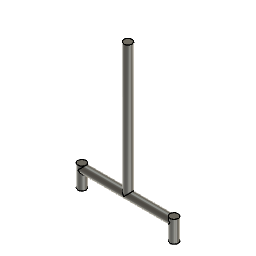
Double-Ended Pendulum v1 (Autodesk Fusion 360 design; units mm, degrees)
Autodesk Fusion 360 part; units mm, degrees
sketch "Sketch1" plane through (0, 0, 0) normal (0, 0, 1) x (1, 0, 0)
  circle A0 centre (-180, 0) radius 8
  circle A1 centre (0, 0) radius 8
  dimension "d1" = 16
  dimension "d2" = 16
  dimension "d3" = 180
  constraint coincident A1.centre origin
  measures "d1" diameter of A0
  measures "d2" diameter of A1
  measures "d3" distance of A0.centre A1.centre
extrude "Extrude1" add sketch "Sketch1" along normal blind 42 makes body 1 at (-172.0099, -0.3988, 28) makes body 2 at (7.9901, -0.3988, 28)
sketch "Sketch2" plane through (0, 0, 0) normal (1, 0, 0) x (0, 1, 0)
  line L0 (8, 42) -> (-8, 42)
  line L1 (8, 0) -> (-8, 0)
  line L2 (0, 42) -> (0, 34) construction
  circle A0 centre (0, 34) radius 8
  dimension "d6" = 8
  constraint midpoint L0 L2.start
  constraint perpendicular L0 L2
  constraint coincident L2.end A0.centre
  constraint coincident L2.start A0
  measures "d6" distance of L2.start L2.end
extrude "Extrude2" add sketch "Sketch2" against normal blind 180 bodies 1 2
ref_plane "WorkPlane1" through (-100.4607, 0, 42) normal (0, 0, 1) x (0, -1, 0)
sketch "Sketch3" plane through (-100.4607, 0, 42) normal (0, 0, 1) x (1, 0, 0)
  arc A0 (-71.5393, 0) -> (-79.5393, 8) centre (-79.5393, 0) ccw
  arc A1 (-79.5393, -8) -> (-71.5393, 0) centre (-79.5393, 0) ccw
  arc A2 (-79.5393, -8) -> (-79.5393, 8) centre (-79.5393, 0) ccw
  arc A3 (100.4607, 8) -> (100.4607, -8) centre (100.4607, 0) ccw
  arc A4 (92.4607, 0) -> (100.4607, -8) centre (100.4607, 0) ccw
  arc A5 (100.4607, 8) -> (92.4607, 0) centre (100.4607, 0) ccw
  circle A6 centre (100.4607, 0) radius 8
  circle A7 centre (-79.5393, 0) radius 8
  line L0 (-79.5393, 0) -> (10.4607, 0) construction
  circle A8 centre (10.4607, 0) radius 8
  dimension "d10" = 90
  dimension "d11" = 16
  constraint coincident A0.centre A1.centre
  constraint horizontal L0
  constraint coincident L0.end A8.centre
  measures "d10" distance of A0.centre L0.end
  measures "d11" diameter of A8
extrude "Extrude3" add sketch "Sketch3" against normal blind 8 contours A8 bodies 1
extrude "Extrude4" add 1 faces at (-92.292, 0.3187, 42) along direction (0, 0, 1) blind 250 on bodies 1 bodies 1
